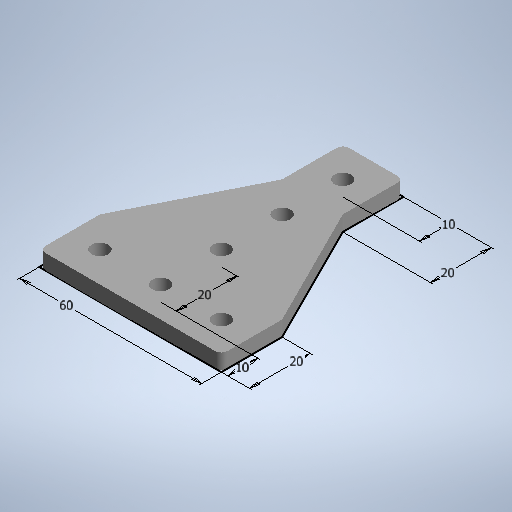
# Autodesk Inventor part: 8060T
Saved by Autodesk Inventor 2025.4 (Build 294407000, 407)
## iProperties
Created: 2026-07-08
Part Number: 8060T
Material: Générique
Document SubType Name: Modeling
Designer: louis
Density: 1 g/cm^3
Appearance: Par défaut
Author: louis
Autodesk Inventor part; units mm, degrees
ref_plane "YZ Plane" through (0, 0, 0) normal (1, 0, 0) x (0, 1, 0)
ref_plane "XZ Plane" through (0, 0, 0) normal (0, 1, 0) x (-1, 0, 0)
ref_plane "XY Plane" through (0, 0, 0) normal (0, 0, 1) x (1, 0, 0)
sketch "Sketch2" plane through (0, 0, 0) normal (0, 0, 1) x (1, 0, 0)
  line L0 (0, 0) -> (0, 20) construction
  line L1 (0, 20) -> (0, 40) construction
  line L2 (0, 40) -> (0, 60) construction
  line L3 (0, 0) -> (20, 0) construction
  line L4 (0, 0) -> (-20, 0) construction
  line L5 (-30, 10) -> (-10, 50)
  line L6 (-10, 50) -> (-10, 70)
  line L7 (-10, 70) -> (10, 70)
  line L8 (10, 70) -> (10, 50)
  line L9 (10, 50) -> (30, 10)
  line L10 (30, 10) -> (30, -10)
  line L11 (30, -10) -> (-30, -10)
  line L12 (-30, -10) -> (-30, 10)
  line L13 (0, 0) -> (0, -10) construction
  line L14 (0, 70) -> (0, 60) construction
  dimension "d0" = 20
  dimension "d1" = 10
  dimension "d2" = 20
  dimension "d3" = 60
  dimension "d4" = 10
  dimension "d5" = 20
  constraints: 30 end point, 7 equal length, 6 coincident, 4 vertical, 3 horizontal, 3 perpendicular, 2 midpoint, 2 point on line, 1 parallel
  measures "d0" distance of L0.start L0.end
  measures "d1" distance of L13.start L13.end
  measures "d2" distance of L9.end L10.end
  measures "d3" distance of L10.end L11.end
  measures "d4" distance from line of L7 L14.end
  measures "d5" distance of L7.end L8.end
extrude "Extrusion1" add sketch "Sketch2" along normal blind 5
hole "Hole1" at (0, 40, 0) at (0, 20, 0) at (0, 60, 0) at (-20, 0, 0) at (0, 0, 0) at (20, 0, 0) direction (0, 0, 1) diameter 5.5 end through all clearance for "Flat Head Machine Screw" size "M5" standard "Ansi Metric M Profile"
fillet "Fillet1" radius 2 8 edges at (-10, 70, 2.5) (-30, 10, 2.5) (-30, -10, 2.5) (30, -10, 2.5) (30, 10, 2.5) (10, 70, 2.5) (10, 50, 2.5) (-10, 50, 2.5)
body "Solid1"
